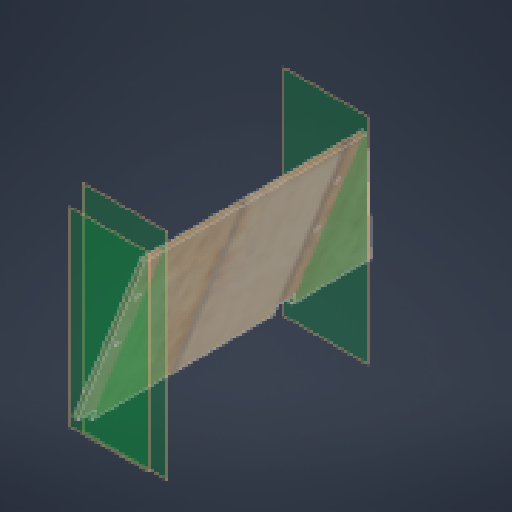
# Autodesk Inventor part: lefft_wall
Saved by Autodesk Inventor 2026.3 (Build 303398000, 398)
## iProperties
Created: 2026-09-07
Part Number: lefft_wall
Material: 木材 (カエデ材)
Document SubType Name: Modeling
Designer: takuya
Density: 0.67 g/cm^3
Appearance: ナチュラル カエデ材 - 光沢 濃い着色
Author: takuya
Autodesk Inventor part; units mm, degrees
ref_plane "YZ Plane" through (0, 0, 0) normal (1, 0, 0) x (0, 1, 0)
ref_plane "作業平面1" through (14.25, -85.0419, 0) normal (0, 0, -1) x (0, 1, 0)
sketch "スケッチ1" plane through (14.25, -85.0419, 0) normal (0, 0, -1) x (0, 1, 0)
  line L0 (-46.6818, -19.75) -> (47.5988, 17.4243) projected
  line L1 (47.5988, 17.4243) -> (46.6818, 19.75) projected
  line L2 (46.6818, 19.75) -> (-47.5988, -17.4243) projected
  line L3 (-47.5988, -17.4243) -> (-46.6818, -19.75) projected
  point P0 (85.0419, -14.25)
ref_plane "作業平面2" through (-8.85, -128.1353, -159.8711) normal (0, 0.3826834, -0.9238795) x (0, 0.9238795, 0.3826834)
extrude "押し出し1" add sketch "スケッチ1" along normal up to surface surface through (-8.85, -128.1353, -159.8711) normal (0, 0.3826834, -0.9238795)
sketch "スケッチ2" plane through (-3.1743, -132.6408, 0) normal (0.930296, -0.3668097, 0) x (0, 0, -1)
  line L0 (0, 30.3562) -> (10, 30.3562) projected
  line L1 (0, 91.3953) -> (0, 30.3562) projected
  line L2 (10, 91.3953) -> (0, 91.3953) projected
  line L3 (10, 30.3562) -> (10, 91.3953) projected
  line L4 (110.4647, 30.3562) -> (120.4647, 30.3562) projected
  line L5 (110.4647, 91.3953) -> (110.4647, 30.3562) projected
  line L6 (120.4647, 91.3953) -> (110.4647, 91.3953) projected
  line L7 (120.4647, 30.3562) -> (120.4647, 91.3953) projected
  line L8 (110.4647, 30.3562) -> (120.4647, 30.3562) projected
  line L9 (110.4647, 91.3953) -> (110.4647, 30.3562) projected
  line L10 (120.4647, 91.3953) -> (110.4647, 91.3953) projected
  line L11 (120.4647, 30.3562) -> (120.4647, 91.3953) projected
  line L12 (0, 91.3953) -> (10, 91.3953)
  line L13 (10, 91.3953) -> (10, 60.8757)
  line L14 (10, 60.8757) -> (0, 60.8757)
  line L15 (0, 60.8757) -> (0, 91.3953)
  line L16 (10, 60.8757) -> (0, 60.8757)
  line L17 (0, 60.8757) -> (0, 30.3562)
  line L18 (0, 30.3562) -> (10, 30.3562)
  line L19 (10, 30.3562) -> (10, 60.8757)
  line L20 (110.4647, 91.3953) -> (120.4647, 91.3953)
  line L21 (120.4647, 91.3953) -> (120.4647, 60.8757)
  line L22 (120.4647, 60.8757) -> (110.4647, 60.8757)
  line L23 (110.4647, 60.8757) -> (110.4647, 91.3953)
  line L24 (120.4647, 60.8757) -> (110.4647, 60.8757)
  line L25 (110.4647, 60.8757) -> (110.4647, 30.3562)
  line L26 (110.4647, 30.3562) -> (120.4647, 30.3562)
  line L27 (120.4647, 30.3562) -> (120.4647, 60.8757)
  circle A0 centre (5, 45.616) radius 1.5
  circle A1 centre (5, 76.1355) radius 1.5
  circle A2 centre (115.4647, 76.1355) radius 1.5
  circle A3 centre (115.4647, 45.616) radius 1.5
  circle A4 centre (115.4647, 76.1355) radius 1.5 projected
  circle A5 centre (115.4647, 45.616) radius 1.5 projected
  circle A6 centre (5, 76.1355) radius 1.5 projected
  circle A7 centre (5, 45.616) radius 1.5 projected
  circle A8 centre (115.4647, 76.1355) radius 1.5 projected
  circle A9 centre (115.4647, 45.616) radius 1.5 projected
  point P0 (0, 124.5595)
  dimension "d2" = 3
  dimension "d3" = 3
  dimension "d4" = 3
  dimension "d5" = 3
  constraints: 32 end point, 8 parallel, 4 centre point, 4 horizontal, 4 perpendicular, 2 midpoint
  measures "d2" diameter of A0
  measures "d3" diameter of A1
  measures "d4" diameter of A2
  measures "d5" diameter of A3
extrude "押し出し2" cut sketch "スケッチ2" against normal blind 2.5 contours A0 | A1 | A2 | A3
ref_plane "作業平面3" through (13.1229, -86.9061, -10) normal (0, 0, -1) x (0, 1, 0)
sketch "スケッチ3" plane through (13.1229, -86.9061, -10) normal (0, 0, -1) x (0, 1, 0)
  line L0 (-44.8176, -18.6229) -> (-45.7346, -16.2971) projected
  line L1 (-50.8753, -21) -> (-51.7923, -18.6743)
  line L2 (-53.8577, -21) -> (53.8577, -21)
  line L3 (-45.423, -16.1743) -> (-53.8577, -19.5)
  line L4 (-51.7923, -18.6743) -> (-50.8753, -21)
  line L5 (-50.8753, -21) -> (-44.8215, -18.613)
  line L6 (-44.8215, -18.613) -> (-45.7385, -16.2873)
  line L7 (-45.7385, -16.2873) -> (-51.7923, -18.6743)
  point P0 (86.9061, -13.1229)
  point P1 (-51.7884, -18.6841)
  constraints: 14 end point, 2 parallel, 2 perpendicular, 1 horizontal, 1 point on line, 8 other
ref_plane "作業平面4" through (-7.8771, -140.7638, -110.4647) normal (0, 0, 1) x (1, 0, 0)
extrude "押し出し3" add sketch "スケッチ3" along normal up to surface (100.4647 mm away) contours L5 L1 L3 L0
ref_plane "作業平面5" through (13.1229, -86.9061, -120.4647) normal (0, 0, -1) x (0, 1, 0)
sketch "スケッチ4" plane through (13.1229, -86.9061, -120.4647) normal (0, 0, -1) x (0, 1, 0)
  line L0 (-44.8176, -18.6229) -> (-45.7346, -16.2971) projected
  line L1 (-50.8753, -21) -> (-51.7923, -18.6743)
  line L2 (49.4342, 18.5514) -> (-50.8753, -21)
  line L3 (-51.7923, -18.6743) -> (48.5172, 20.8771)
  line L4 (-45.7346, -16.2971) -> (-44.8176, -18.6229)
  line L5 (-44.8176, -18.6229) -> (-50.8714, -21.0098)
  line L6 (-50.8714, -21.0098) -> (-51.7884, -18.6841)
  line L7 (-51.7884, -18.6841) -> (-45.7346, -16.2971)
  point P0 (86.9061, -13.1229)
  point P1 (-51.7884, -18.6841)
  point P2 (-44.8215, -18.613)
  constraints: 14 end point, 2 parallel, 2 perpendicular, 1 point on line, 7 other
extrude "押し出し4" add sketch "スケッチ4" along normal up to surface contours L2 L1 L7 L0 surface through (14.25, -85.0419, -142.0212) normal (0, 0.3826834, -0.9238795)
sketch "スケッチ7" plane through (34, -38.3601, 0) normal (0.930296, -0.3668097, 0) x (0, 0, -1)
  circle A0 centre (5, -55.7288) radius 1.5 projected
  circle A1 centre (115.4647, -55.7288) radius 1.5 projected
  circle A2 centre (5, -25.2093) radius 1.5 projected
  circle A3 centre (115.4647, -25.2093) radius 1.5 projected
  line L0 (164.2448, -107.8521) -> (122.685, 0) projected
  line L1 (0, 0) -> (122.685, 0) projected
  line L2 (0, 0) -> (0, -101.3448) projected
  line L3 (0, -101.3448) -> (10, -101.3448) projected
  line L4 (10, -101.3448) -> (10, -107.8521) projected
  line L5 (10, -107.8521) -> (110.4647, -107.8521) projected
  line L6 (110.4647, -101.3448) -> (110.4647, -107.8521) projected
  line L7 (110.4647, -101.3448) -> (120.4647, -101.3448) projected
  line L8 (120.4647, -101.3448) -> (120.4647, -107.8521) projected
  line L9 (120.4647, -107.8521) -> (164.2448, -107.8521) projected
  line L10 (122.1491, 0) -> (163.709, -107.8521)
  line L11 (164.2448, -107.8521) -> (122.685, 0) projected
  point P0 (0, 23.2147)
  dimension "d13" = 0.5
  constraints: 2 end point, 2 point on line, 1 parallel
  measures "d13" distance between parallel lines of L11 L10
extrude "押し出し5" cut sketch "スケッチ7" against normal blind 2.5 contours L9 L10 L1 L0
